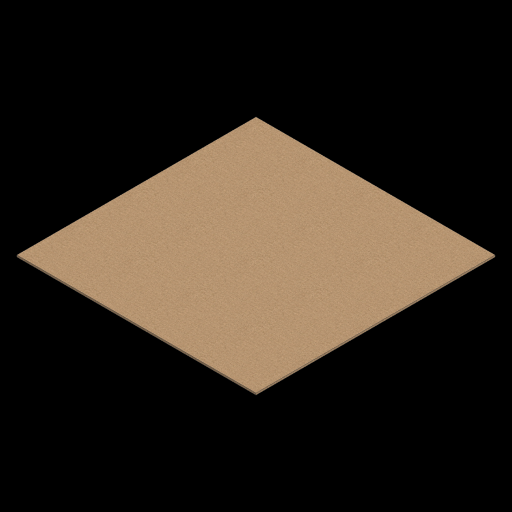
# Autodesk Inventor part: C41x41
Saved by Autodesk Inventor 2024.2 (Build 282272000, 272)
## iProperties
Created: 2024-07-18
Part Number: C41x41
Material: MDF Medium Density Fiberboard
Document SubType Name: Modeling
Designer: jrcer
Density: 0.8 g/cm^3
Appearance: Cardboard - Corrugated
Author: jrcer
Autodesk Inventor part; units mm, degrees
ref_plane "YZ Plane" through (0, 0, 0) normal (1, 0, 0) x (0, 1, 0)
ref_plane "XZ Plane" through (0, 0, 0) normal (0, 1, 0) x (-1, 0, 0)
ref_plane "XY Plane" through (0, 0, 0) normal (0, 0, 1) x (1, 0, 0)
sketch "Sketch1" plane through (0, 0, 0) normal (0, 1, 0) x (-1, 0, 0)
  line L0 (210, 210) -> (-210, 210)
  line L1 (-210, 210) -> (-210, -210)
  line L2 (-210, -210) -> (210, -210)
  line L3 (210, -210) -> (210, 210)
  line L4 (210, 210) -> (-210, -210) construction
  line L5 (-210, 210) -> (210, -210) construction
  point P0 (0, 0)
  dimension "d0" = 420
  dimension "d1" = 420
  constraints: 12 end point, 2 midpoint, 2 parallel, 1 horizontal, 1 perpendicular
  measures "d0" distance of L2.end L1.end
  measures "d1" distance of L1.end L0.end
extrude "Extrusion1" add sketch "Sketch1" along normal blind 3.25
sketch "Sketch2" plane through (0, 3.25, 0) normal (0, 1, 0) x (1, 0, 0)
  line L0 (-10, -55) -> (10, -55)
  line L1 (10, -55) -> (10, -60)
  line L2 (10, -60) -> (-10, -60)
  line L3 (-10, -60) -> (-10, -55)
  point P0 (0, 0)
  point P1 (0, -60)
  dimension "d4" = 20
  dimension "d5" = 5
  dimension "d6" = 60
  constraints: 8 end point, 2 parallel, 1 horizontal, 1 midpoint, 1 perpendicular, 1 vertical alignment
  measures "d4" distance of L1.end L2.end
  measures "d5" distance between parallel lines of L2 L0
  measures "d6" distance from line of L2 point (0, 0)
extrude "Extrusion2" [suppressed]
sketch "Sketch3" plane through (0, 3.25, 0) normal (0, 1, 0) x (1, 0, 0)
  line L0 (210, -210) -> (210, 210) construction
  line L1 (210, 210) -> (-210, 210) construction
  line L2 (-210, 210) -> (-210, -210) construction
  line L3 (-210, -210) -> (210, -210) construction
  line L4 (-200, 200) -> (200, 200)
  line L5 (200, 200) -> (200, -200)
  line L6 (200, -200) -> (-200, -200)
  line L7 (-200, -200) -> (-200, 200)
  line L8 (-200, 200) -> (200, -200) construction
  line L9 (200, 200) -> (-200, -200) construction
  point P0 (0, 0)
  dimension "d9" = 400
  dimension "d10" = 400
  constraints: 12 end point, 2 midpoint, 2 parallel, 1 horizontal, 1 perpendicular
  measures "d9" distance of L5.end L6.end
  measures "d10" distance of L4.end L5.end
body "Solid1"
